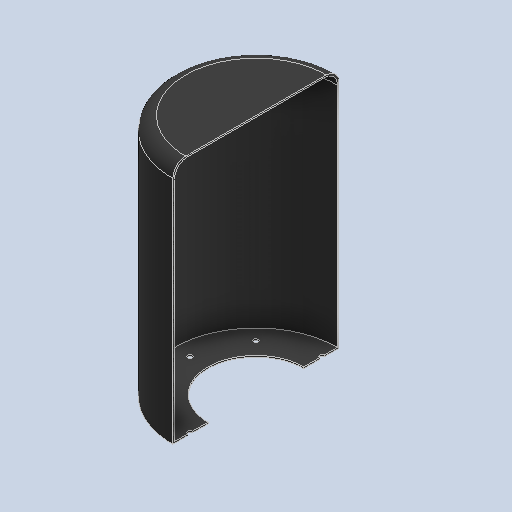
# Autodesk Inventor part: Capa
Saved by Autodesk Inventor 2025.3 (Build 293356030, 356C)
## iProperties
Created: 2025-10-13
Part Number: Capa
Material: Caucho, Silicona
Document SubType Name: Modeling
Designer: santa
Density: 1.25 g/cm^3
Appearance: Caucho - Negro
Author: santa
Autodesk Inventor part; units mm, degrees
ref_plane "YZ Plane" through (0, 0, 0) normal (1, 0, 0) x (0, 1, 0)
ref_plane "XZ Plane" through (0, 0, 0) normal (0, 1, 0) x (-1, 0, 0)
ref_plane "XY Plane" through (0, 0, 0) normal (0, 0, 1) x (1, 0, 0)
sketch "Boceto1" plane through (0, 0, 0) normal (0, 1, 0) x (-1, 0, 0)
  circle A0 centre (0, 0) radius 51
  circle A1 centre (0, 0) radius 30
  circle A2 centre (0, 0) radius 52
  point P0 (41.233, 0)
  point P1 (29.1561, 29.1561)
  point P2 (0, 41.233)
  point P3 (-29.1561, 29.1561)
  point P4 (-41.233, 0)
  point P5 (-29.1561, -29.1561)
  point P6 (0, -41.233)
  point P7 (29.1561, -29.1561)
  dimension "d0" = 102
  dimension "d1" = 60
  dimension "d2" = 41.233
  dimension "d3" = 1
  dimension "d8" = 360
  constraints: 3 centre point, 2 coincident, 1 horizontal alignment, 9 other
  measures "d0" diameter of A0
  measures "d1" diameter of A1
  measures "d2" distance of point (0, 0) point (41.233, 0)
  measures "d3" radial gap between concentric circles of A0 A2
extrude "Extrusión1" add sketch "Boceto1" along normal blind 1 contours A0
extrude "Extrusión2" add sketch "Boceto1" along normal blind 152 contours A0 | A2
sketch "Boceto3" plane through (0, 152, 0) normal (0, 1, 0) x (1, 0, 0)
  circle A0 centre (0, 0) radius 30 projected
extrude "Extrusión4" add sketch "Boceto3" against normal blind 151
shell "Vaciado1" thickness 1 removed faces 1 at (-8.8546, 1, 4.6472)
fillet "Empalme1" radius 8 2 edges at (51, 151, 0) (52, 152, 0)
hole "Hole1" at (-41.233, 0, 0) at (-29.1561, 0, 29.1561) at (0, 0, 41.233) at (29.1561, 0, 29.1561) at (41.233, 0, 0) at (29.1561, 0, -29.1561) at (0, 0, -41.233) at (-29.1561, 0, -29.1561) direction (0, 1, 0) diameter 3 depth 8 tip angle 118
